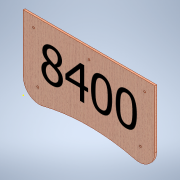
# Autodesk Inventor part: FTC Outside Panels
Saved by Autodesk Inventor 2020 (Build 240168000, 168)
## iProperties
Created: 2022-09-23
Part Number: FTC Outside Panels
Material: Wood (Oak)
Document SubType Name: Modeling
Designer: Jason
Density: 0.76 g/cm^3
Appearance: White Oak - Natural Medium Gloss
Author: Jason
Autodesk Inventor part; units mm, degrees
ref_plane "YZ Plane" through (0, 0, 0) normal (1, 0, 0) x (0, 1, 0)
ref_plane "XZ Plane" through (0, 0, 0) normal (0, 1, 0) x (-1, 0, 0)
ref_plane "XY Plane" through (0, 0, 0) normal (0, 0, 1) x (1, 0, 0)
sketch "Sketch1" plane through (0, 0, 0) normal (0, 0, 1) x (1, 0, 0)
  line L0 (49.2125, 0) -> (54.6328, 0)
  line L1 (357.1875, 0) -> (350.9902, 0)
  arc A0 (0, 49.2125) -> (65.0875, 2.6308) centre (49.2125, 49.2125) ccw
  arc A1 (345.2239, 1.4763) -> (406.4, 49.2125) centre (357.1875, 49.2125) ccw
  arc A2 (203.2, 19.05) -> (54.6328, 0) centre (202.8115, -566.7686) ccw
  arc A3 (350.9902, 0) -> (345.2239, 1.4763) centre (202.8115, -566.7686) ccw
  arc A4 (65.0875, 2.6308) -> (54.6328, 0) centre (202.8115, -566.7686) ccw
  arc A5 (350.9902, 0) -> (203.2, 19.05) centre (202.8115, -566.7686) ccw
  line L2 (0, 49.2125) -> (0, 228.6)
  line L3 (406.4, 228.6) -> (406.4, 49.2125)
  line L4 (0, 228.6) -> (406.4, 228.6)
  point P0 (0, 0)
  point P1 (57.0671, 0.6309)
  constraints: 16 point on circle, 10 end point, 6 centre point, 1 perpendicular, 1 vertical
extrude "Extrusion1" add sketch "Sketch1" along normal blind 5.5563 contours A0 L2 L4 L3 A1 A5 A2
sketch "Sketch5" plane through (0, 0, 5.5563) normal (0, 0, 1) x (1, 0, 0)
  line L0 (51.1152, 176.6695) -> (357.0209, 176.6695) construction
  line L1 (357.0209, 176.6695) -> (357.0209, 65.074) construction
  line L2 (357.0209, 65.074) -> (51.1152, 65.074) construction
  line L3 (51.1152, 65.074) -> (51.1152, 176.6695) construction
  point P0 (0, 0)
  constraints: 2 other
sketch "Sketch6" plane through (0, 0, 5.5563) normal (0, 0, 1) x (1, 0, 0)
  line L0 (406.4, 228.6) -> (0, 228.6)
  line L1 (0, 228.6) -> (0, 49.2125)
  circle A0 centre (31.75, 196.85) radius 2.9337
  line L2 (406.4, 49.2125) -> (406.4, 228.6)
  circle A1 centre (374.65, 196.85) radius 2.9337
  circle A2 centre (203.2, 196.85) radius 2.9337
  arc A3 (345.2239, 1.4763) -> (406.4, 49.2125) centre (357.1875, 49.2125) ccw
  circle A4 centre (361.7391, 44.6609) radius 2.9337
  arc A5 (0, 49.2125) -> (57.0671, 0.6309) centre (49.2125, 49.2125) ccw
  circle A6 centre (44.6609, 44.6609) radius 2.9337
  point P0 (0, 0)
  point P1 (0, 0)
  constraints: 7 centre point, 6 end point, 4 point on circle
extrude "Extrusion6" cut sketch "Sketch6" against normal up to surface (5.5563 mm away)
body "Solid1"
